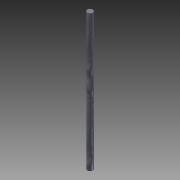
# Autodesk Inventor part: Shaft 80mm
Saved by Autodesk Inventor 2015 (Build 190159000, 159)
## iProperties
Created: 2013-10-24
Part Number: Shaft 80mm
Material: ステンレス鋼 AISI 440C、溶接
Document SubType Name: Modeling
Designer: kenta
Density: 7.8 g/cm^3
Appearance: 溶接 - ステンレス鋼
Mass: 2.82291 g
Surface Area: 4.96686 cm^2
Volume: 0.361911 cm^3
Author: kenta
Autodesk Inventor part; units mm, degrees
ref_plane "YZ Plane" through (0, 0, 0) normal (1, 0, 0) x (0, 1, 0)
ref_plane "XZ Plane" through (0, 0, 0) normal (0, 1, 0) x (-1, 0, 0)
ref_plane "XY Plane" through (0, 0, 0) normal (0, 0, 1) x (1, 0, 0)
sketch "スケッチ1" plane through (0, 0, 0) normal (0, 0, 1) x (1, 0, 0)
  circle A0 centre (0, 0) radius 1.5
  dimension "d0" = 3
  constraints: 1 centre point, 1 coincident
  measures "d0" diameter of A0
extrude "押し出し1" add sketch "スケッチ1" along normal blind 75
